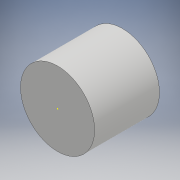
# Autodesk Inventor part: 伸縮缸 球軸 座
Saved by Autodesk Inventor 2017 (Build 210142000, 142)
## iProperties
Part Number: 伸縮缸 球軸 座
Material: 一般
Document SubType Name: Modeling
Designer: NB23-1
Density: 1 g/cm^3
Appearance: 預設
Author: NB23-1
Autodesk Inventor part; units mm, degrees
ref_plane "YZ Plane" through (0, 0, 0) normal (1, 0, 0) x (0, 1, 0)
ref_plane "XZ Plane" through (0, 0, 0) normal (0, 1, 0) x (-1, 0, 0)
ref_plane "XY Plane" through (0, 0, 0) normal (0, 0, 1) x (1, 0, 0)
sketch "草圖1" plane through (0, 0, 0) normal (0, 0, 1) x (1, 0, 0)
  arc A0 (0, -5.4) -> (0, 5.4) centre (0, 0) ccw
  line L0 (0, 0) -> (0, -5.4) construction
  line L1 (0, 0) -> (0, 5.4) construction
  line L2 (0, -5.4) -> (0, -10.4)
  line L3 (0, -10.4) -> (8, -10.4)
  line L4 (8, -10.4) -> (8, 3.6)
  line L5 (8, 3.6) -> (4.0249, 3.6)
  dimension "d0" = 5.4
  dimension "d1" = 180
  dimension "d2" = 5
  dimension "d3" = 8
  dimension "d4" = 14
  constraints: 12 end point, 3 point on circle, 2 perpendicular, 1 centre point, 1 coincident, 1 horizontal, 1 vertical
  measures "d0" radius of A0
  measures "d1" angle of L0 L1
  measures "d2" distance of L0.end L2.end
  measures "d3" distance of L2.end L3.end
  measures "d4" distance of L3.end L4.end
revolve "迴轉1" add sketch "草圖1" angle 360 about axis through (0, -5.4, 0) along (0, -1, 0)
sketch "草圖2" plane through (0, -10.4, 0) normal (0, -1, 0) x (1, 0, 0)
  point P0 (0, 0)
